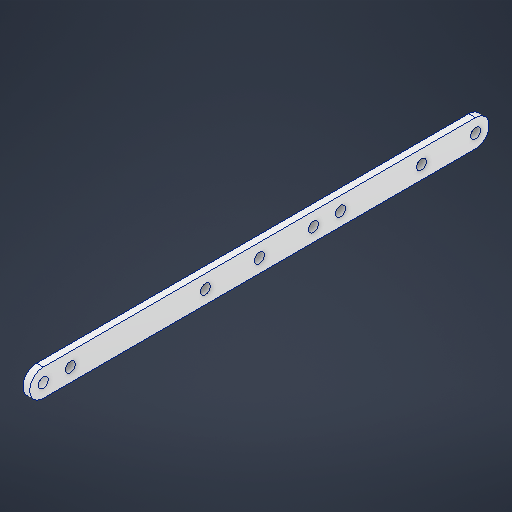
# Autodesk Inventor part: Conveyor chassis
Saved by Autodesk Inventor 2025 (Build 290162000, 162)
## iProperties
Created: 2024-12-28
Part Number: Conveyor chassis
Material: Aluminum 6061
Document SubType Name: Sheet Metal
Designer: Juan
Density: 2.7 g/cm^3
Sheet Metal Rule: Default
Appearance: Aluminum - Flat
Author: Juan
Autodesk Inventor part; units mm, degrees
ref_plane "YZ Plane" through (0, 0, 0) normal (1, 0, 0) x (0, 1, 0)
ref_plane "XZ Plane" through (0, 0, 0) normal (0, 1, 0) x (-1, 0, 0)
ref_plane "XY Plane" through (0, 0, 0) normal (0, 0, 1) x (1, 0, 0)
sketch "Sketch1" plane through (0, 0, 0) normal (1, 0, 0) x (0, 1, 0)
  line L0 (0, 0) -> (0, -203.2) construction
  line L1 (-6.35, 0) -> (-6.35, -203.2)
  line L2 (6.35, -203.2) -> (6.35, 0)
  arc A0 (6.35, 0) -> (-6.35, 0) centre (0, 0) ccw
  arc A1 (-6.35, -203.2) -> (6.35, -203.2) centre (0, -203.2) ccw
  circle A2 centre (0, 0) radius 2.3241
  circle A3 centre (0, -203.2) radius 2.3241
  line L3 (0, 0) -> (0, -12.7)
  circle A4 centre (0, -12.7) radius 2.3241
  line L4 (0, -12.7) -> (0, -76.2)
  circle A5 centre (0, -76.2) radius 2.3241
  line L5 (0, -76.2) -> (0, -101.6)
  circle A6 centre (0, -101.6) radius 2.3241
  line L6 (0, -101.6) -> (0, -127)
  circle A7 centre (0, -127) radius 2.3241
  line L7 (0, -127) -> (0, -177.8)
  circle A8 centre (0, -177.8) radius 2.3241
  line L8 (0, -12.7) -> (0, -38.1)
  line L9 (-6.35, -38.1) -> (6.35, -38.1)
  line L10 (0, -127) -> (0, -139.7)
  circle A9 centre (0, -139.7) radius 2.3241
  dimension "d0" = 203.2
  dimension "d1" = 12.7
  dimension "d2" = 4.6482
  dimension "d3" = 4.6482
  dimension "d4" = 12.7
  dimension "d5" = 63.5
  dimension "d6" = 4.6482
  dimension "d7" = 25.4
  dimension "d8" = 4.6482
  dimension "d9" = 25.4
  dimension "d10" = 4.6482
  dimension "d11" = 50.8
  dimension "d12" = 4.6482
  dimension "d14" = 25.4
  dimension "d15" = 12.7
  dimension "d16" = 4.6482
  measures "d0" distance of L1.start L1.end
  measures "d1" distance of L2.start L1.end
  measures "d2" diameter of A2
  measures "d3" diameter of A3
  measures "d4" distance of L3.start L3.end
  measures "d5" distance of L4.start L4.end
  measures "d6" diameter of A5
  measures "d7" distance of L5.start L5.end
  measures "d8" diameter of A6
  measures "d9" distance of L6.start L6.end
  measures "d10" diameter of A7
  measures "d11" distance of L7.start L7.end
  measures "d12" diameter of A8
  measures "d14" distance of L4.start L8.end
  measures "d15" distance of L7.start L10.end
  measures "d16" diameter of A9
extrude "Plate1" add sketch "Sketch1" along normal blind 3.175 contours A0 L2 L9 L1 | L9 L2 A1 L1 | A9 L7 | L7 A9
sketch "Sketch2" plane through (3.175, 0, 0) normal (1, 0, 0) x (0, 0, -1)
  circle A0 centre (127, 0) radius 2.3241 projected
  line L0 (127, 0) -> (139.7, 0)
  circle A1 centre (139.7, 0) radius 2.3241
  point P0 (0, 0)
  dimension "d17" = 12.7
  dimension "d18" = 4.6482
  constraints: 2 end point, 1 centre point, 1 coincident, 1 horizontal
  measures "d17" distance of L0.start L0.end
  measures "d18" diameter of A1
extrude "Cut1" cut sketch "Sketch2" against normal blind 3.175 contours A1
equation "\"d19\" = Thickness"
equation "\"d13\" = Thickness"
equation "\"BendRadius\" = Thickness"
equation "\"BendReliefWidth\" = Thickness"
equation "\"BendReliefDepth\" = 0.5 * Thickness"
equation "\"CornerReliefSize\" = 4 * Thickness"
equation "\"MinimumRemnant\" = 2 * Thickness"
equation "\"TransitionRadius\" = BendRadius"
equation "\"JacobiRadiusSize\" = BendRadius"
equation "\"GapSize\" = Thickness"
equation "\"Thickness\" = 3.175"
body "Solid1"
